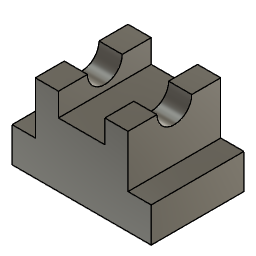
Lesson2 v0 (Autodesk Fusion 360 design; units mm, degrees)
Autodesk Fusion 360 part; units mm, degrees
sketch "Sketch1" plane through (0, 0, 0) normal (0, 1, 0) x (1, 0, 0)
  line L0 (60, 15) -> (-60, 15)
  line L1 (-60, 15) -> (-60, -15)
  line L2 (-60, -15) -> (60, -15)
  line L3 (60, -15) -> (60, 15)
  line L4 (60, 15) -> (-60, -15) construction
  line L5 (-60, 15) -> (60, -15) construction
  line L6 (0, -15) -> (0, -60)
  line L7 (40, -15) -> (-40, -15)
  line L8 (-40, -15) -> (-40, -60)
  line L9 (-40, -60) -> (40, -60)
  line L10 (40, -60) -> (40, -15)
  line L11 (40, -15) -> (-40, -60) construction
  line L12 (-40, -15) -> (40, -60) construction
  line L13 (20, -40) -> (-20, -40)
  line L14 (-20, -40) -> (-20, -80)
  line L15 (-20, -80) -> (20, -80)
  line L16 (20, -80) -> (20, -40)
  line L17 (20, -40) -> (-20, -80) construction
  line L18 (-20, -40) -> (20, -80) construction
  point P0 (0, -37.5)
  point P1 (0, -60)
  dimension "d1" = 120
  dimension "d2" = 30
  dimension "d3" = 45
  dimension "d4" = 80
  dimension "d5" = 40
  dimension "d6" = 40
  constraint horizontal L0
  constraint perpendicular L0 L1
  constraint parallel L0 L2
  constraint parallel L1 L3
  constraint coincident L4 origin
  constraint coincident L5 origin
  constraint midpoint L2 L6.start
  constraint perpendicular L2 L6
  constraint horizontal L7
  constraint perpendicular L7 L8
  constraint parallel L7 L9
  constraint parallel L8 L10
  constraint coincident L11 P0
  constraint coincident L12 P0
  constraint midpoint L6 P0
  constraint horizontal L13
  constraint perpendicular L13 L14
  constraint parallel L13 L15
  constraint parallel L14 L16
  constraint coincident L17 P1
  constraint coincident L18 P1
  constraint coincident P1 L6.end
  measures "d1" distance of L1.end L2.end
  measures "d2" distance of L0.end L1.end
  measures "d3" distance of L6.start P1
  measures "d4" distance of L8.end L9.end
  measures "d5" distance of L14.end L15.end
  measures "d6" distance of L13.end L14.end
extrude "Extrude1" add sketch "Sketch1" along normal blind 80 contours L0 L1 L2 L3 L7 | L2 L6 L7 L9 L10 L13 L16 | L2 L6 L7 L8 L9 L13 L14
sketch "Sketch2" plane through (40, 0, 0) normal (1, 0, 0) x (0, 1, 0)
  line L0 (0, 60) -> (0, 15)
  line L1 (0, 15) -> (80, 15)
  line L2 (80, 15) -> (80, 60)
  line L3 (80, 60) -> (0, 60)
  circle A0 centre (40, 60) radius 15
  dimension "d9" = 30
  constraint midpoint L3 A0.centre
  measures "d9" diameter of A0
extrude "Extrude2" cut sketch "Sketch2" against normal blind 100 contours L3 A0 | L3 A0
